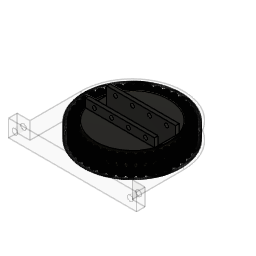
Fiber_stretcher_rotating_mount v3 (Autodesk Fusion 360 design; units mm, degrees)
Autodesk Fusion 360 part; units mm, degrees
note: some values were not read from the file. Set by a fixed rule: which sketch regions a step uses.
other "Base Mesh Feature1"
other "CutPasteMeshes1" in component "Bearing"
sketch "Sketch1" plane through (0, 0, 0) normal (0, 0, 1) x (1, 0, 0) in component "Outer_mount"
  circle A0 centre (0, 0) radius 56.5
  circle A1 centre (0, 0) radius 60
  line L0 (-75, -60) -> (75, -60)
  line L1 (-75, -70) -> (75, -70)
  line L2 (-75, -60) -> (-75, -70)
  line L3 (75, -60) -> (75, -70)
  line L4 (-60, -60) -> (-60, 0)
  line L5 (60, 0) -> (60, -60)
  dimension "d8" = 113
  dimension "d10" = 120
  dimension "d11" = 150
  dimension "d12" = 75
  dimension "d13" = 150
  dimension "d14" = 10
  constraint coincident A0.centre A1.centre
  constraint horizontal L0
  constraint tangent A1 L0
  constraint horizontal L1
  constraint perpendicular L1 L2
  constraint coincident L0 L4.start
  constraint coincident A1 L4.end
  constraint coincident A1 L5.start
  constraint coincident L0 L5.end
  constraint perpendicular L0 L5
  constraint perpendicular L0 L4
  constraint tangent A1 L4
  constraint tangent A1 L5
  measures "d8" diameter of A0
  measures "d10" diameter of A1
  measures "d11" distance of L0.start L0.end
  measures "d12" horizontal distance of A0.centre L0.end
  measures "d13" distance of L1.start L1.end
  measures "d14" distance of L0 L1
other "Scale1" in component "Bearing"
extrude "Extrude1" add sketch "Sketch1" along normal blind 20 makes body 1 in component "Outer_mount"
other "Modify1" in component "Bearing"
sketch "Sketch2" plane through (0, -60, 0) normal (0, 1, 0) x (-1, 0, 0) in component "Outer_mount"
  line L0 (60, 0) -> (75, 0)
  line L1 (75, 0) -> (75, 20)
  line L2 (75, 20) -> (60, 20)
  line L3 (60, 20) -> (60, 0)
  circle A0 centre (67.5, 10) radius 3.25
  circle A1 centre (-67.5, 10) radius 3.25
  line L4 (-60, 0) -> (-75, 0)
  line L5 (-75, 0) -> (-75, 20)
  dimension "d20" = 6.5
  dimension "d21" = 10
  dimension "d22" = 10
  dimension "d23" = 7.5
  dimension "d24" = 7.5
  constraint equal A0 A1
  measures "d20" diameter of A1
  measures "d21" distance of A1.centre L4
  measures "d22" distance of L0 A0.centre
  measures "d23" distance of L1 A0.centre
  measures "d24" distance of A1.centre L5
extrude "Extrude2" cut sketch "Sketch2" against normal through all contours A0 | A1 bodies 1 in component "Outer_mount"
sketch "Sketch1 (2)" plane through (0, 0, 0) normal (0, 0, 1) x (1, 0, 0) in component "Inner_mount"
  circle A0 centre (0, 0) radius 43
  line L0 (-40.5, 10.25) -> (40.5, 10.25)
  line L1 (40.5, 10.25) -> (40.5, -10.25)
  line L2 (40.5, -10.25) -> (-40.5, -10.25)
  line L3 (-40.5, -10.25) -> (-40.5, 10.25)
  dimension "d34" = 86
  dimension "d35" = 81
  dimension "d36" = 40.5
  dimension "d37" = 10.25
  dimension "d38" = 20.5
  constraint coincident A0.centre origin
  constraint horizontal L0
  constraint vertical L1
  constraint horizontal L2
  constraint vertical L3
  measures "d34" diameter of A0
  measures "d35" distance of L0.start L0.end
  measures "d36" distance of A0.centre L3
  measures "d37" vertical distance of A0.centre L0.start
  measures "d38" distance of L0.start L2.end
extrude "Extrude1'" add sketch "Sketch1 (2)" along normal blind 20 separate body makes body 2 in component "Inner_mount"
sketch "Sketch2 (2)" plane through (0, 0, 20) normal (0, 0, 1) x (-1, 0, 0) in component "Inner_mount"
  line L0 (-40.5, 10.25) -> (40.5, 10.25)
  line L1 (40.5, 10.25) -> (40.5, -10.25)
  line L2 (40.5, -10.25) -> (-40.5, -10.25)
  line L3 (-40.5, -10.25) -> (-40.5, 10.25)
  circle A0 centre (0, 0) radius 43
  line L4 (-40.5, 10.25) -> (40.5, 10.25)
  line L5 (40.5, 10.25) -> (40.5, 14.4482)
  line L6 (40.5, 14.4482) -> (-40.5, 14.4482)
  line L7 (-40.5, 14.4482) -> (-40.5, 10.25)
  line L8 (-40.5, -10.25) -> (40.5, -10.25)
  line L9 (40.5, -10.25) -> (40.5, -14.4482)
  line L10 (40.5, -14.4482) -> (-40.5, -14.4482)
  line L11 (-40.5, -14.4482) -> (-40.5, -10.25)
  constraint horizontal L4
  constraint vertical L5
  constraint horizontal L6
  constraint vertical L7
  constraint coincident L0.start L3.end
  constraint horizontal L8
  constraint vertical L9
  constraint horizontal L10
  constraint vertical L11
  constraint coincident A0 L9.end
  constraint coincident L2.end L3.start
  constraint coincident L1.end L9
  constraint coincident L0.end L5
  constraint coincident A0 L6.end
extrude "Extrude2'" add sketch "Sketch2 (2)" along normal blind 10 contours L0 L4 L5 L6 L7 | L2 L8 L9 L10 L11 bodies 2 in component "Inner_mount"
sketch "Sketch3" plane through (0, -14.4482, 0) normal (0, -1, 0) x (1, 0, 0) in component "Inner_mount"
  line L0 (-40.5, 20) -> (40.5, 20)
  line L1 (40.5, 20) -> (40.5, 30)
  line L2 (40.5, 30) -> (-40.5, 30)
  line L3 (-40.5, 30) -> (-40.5, 20)
  circle A0 centre (-30, 25) radius 2.2361
  circle A1 centre (-10, 25) radius 2.2361
  circle A2 centre (10, 25) radius 2.2361
  circle A3 centre (30, 25) radius 2.2361
  line L4 (-48.3551, 25) -> (53.6449, 25)
  dimension "d44" = 5
  dimension "d45" = 20
  dimension "d46" = 20
  dimension "d47" = 20
  dimension "d48" = 10.5
  constraint equal A0 A1
  constraint equal A1 A2
  constraint equal A2 A3
  constraint perpendicular L3 L4
  constraint coincident A0.centre L4
  constraint coincident A1.centre L4
  constraint coincident A2.centre L4
  constraint coincident A3.centre L4
  measures "d44" vertical distance of L2.end L4.start
  measures "d45" distance of A0.centre A1.centre
  measures "d46" distance of A1.centre A2.centre
  measures "d47" distance of A2.centre A3.centre
  measures "d48" horizontal distance of L2.end A0.centre
extrude "Extrude3" cut sketch "Sketch3" against normal through all contours A0 L4 | A0 L4 | A3 L4 | A3 L4 | A1 L4 | A1 L4 | A2 L4 | A2 L4 bodies 2 in component "Inner_mount"
component "Bearing" placed x (1, 0, 0) y (0, 1, 0) z (0, 0, 1) at (0, 0, 0)
component "Outer_mount" placed x (1, 0, 0) y (0, 1, 0) z (0, 0, 1) at (0, 0, 0)
component "Inner_mount" placed x (1, 0, 0) y (0, 1, 0) z (0, 0, 1) at (0, 0, 0)
equation "outer_int_d = 113 mm"
equation "outer_ext_d = 120 mm"
equation "m6_washer_d = 15 mm"
equation "m6_hole = 6.5 mm"
equation "hight = 20 mm"
equation "base_w = outer_ext_d + 2 * m6_washer_d"
equation "base_t = 10 mm"
equation "d8 = outer_int_d"
equation "d10 = outer_ext_d"
equation "d11 = base_w"
equation "d12 = base_w / 2"
equation "d13 = base_w"
equation "d14 = base_t"
equation "d15 = hight"
equation "d19 = hight / 2"
equation "d20 = m6_hole"
equation "d21 = hight / 2"
equation "d22 = hight / 2"
equation "d23 = m6_washer_d / 2"
equation "d24 = m6_washer_d / 2"
equation "profile_w = 81 mm"
equation "profile_t = 20.5 mm"
equation "m4_hole = 5 mm"
equation "profile_holding_plate_t = 5 mm"
equation "profile_holding_plate_h = 10 mm"
equation "hole_spacing = 20 mm"
equation "edge_spacing = 10.5 mm"
equation "inner_out_d = 86 mm"
equation "d34 = inner_out_d"
equation "d35 = profile_w"
equation "d36 = profile_w / 2"
equation "d37 = profile_t / 2"
equation "d38 = profile_t"
equation "d39 = hight"
equation "d42 = profile_holding_plate_h"
equation "d44 = profile_holding_plate_h / 2"
equation "d45 = hole_spacing"
equation "d46 = hole_spacing"
equation "d47 = hole_spacing"
equation "d48 = edge_spacing"
